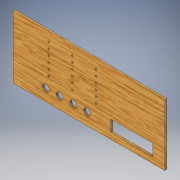
# Autodesk Inventor part: wooden-panel
Saved by Autodesk Inventor 2019.2 (Build 232265000, 265)
## iProperties
Created: 2020-05-18
Part Number: wooden-panel
Material: Laminated Veneer Lumber
Document SubType Name: Modeling
Designer: Johansson
Density: 0.51 g/cm^3
Appearance: Plywood - New
Author: Johansson
Autodesk Inventor part; units mm, degrees
ref_plane "YZ Plane" through (0, 0, 0) normal (1, 0, 0) x (0, 1, 0)
ref_plane "XZ Plane" through (0, 0, 0) normal (0, 1, 0) x (-1, 0, 0)
ref_plane "XY Plane" through (0, 0, 0) normal (0, 0, 1) x (1, 0, 0)
sketch "Sketch1" plane through (0, 0, 0) normal (0, 0, 1) x (1, 0, 0)
  line L0 (0, 0) -> (640, 0)
  line L1 (640, 0) -> (640, 260)
  line L2 (640, 260) -> (0, 265)
  line L3 (0, 265) -> (0, 0)
  dimension "d0" = 640
  dimension "d1" = 260
  dimension "d2" = 265
  constraints: 8 end point, 1 horizontal, 1 parallel, 1 perpendicular
  measures "d0" distance of L0.start L0.end
  measures "d1" distance of L0.end L1.end
  measures "d2" distance of L2.end L0.start
extrude "Extrusion1" add sketch "Sketch1" along normal blind 8
sketch "Sketch2" plane through (0, 0, 8) normal (0, 0, 1) x (1, 0, 0)
  line L0 (412, 75) -> (590, 75)
  line L1 (590, 75) -> (590, 25)
  line L2 (590, 25) -> (412, 25)
  line L3 (412, 25) -> (412, 75)
  line L4 (640, 0) -> (640, 260) projected
  line L5 (0, 0) -> (640, 0) projected
  dimension "d5" = 178
  dimension "d6" = 50
  dimension "d7" = 50
  dimension "d8" = 25
  constraints: 8 end point, 2 parallel, 1 horizontal, 1 perpendicular
  measures "d5" distance of L1.end L2.end
  measures "d6" distance of L0.end L1.end
  measures "d7" distance between parallel lines of L1 L4
  measures "d8" distance between parallel lines of L5 L2
extrude "Extrusion2" cut sketch "Sketch2" against normal up to next
sketch "Sketch3" plane through (0, 0, 8) normal (0, 0, 1) x (1, 0, 0)
  circle A0 centre (150, 100) radius 4
  line L0 (150, 314.3416) -> (150, 72.5342) construction
  line L1 (590, 75) -> (590, 25) projected
  line L2 (412, 75) -> (590, 75) projected
  line L3 (0, 265) -> (0, 0) projected
  dimension "d11" = 8
  dimension "d13" = 25
  dimension "d36" = 150
  constraints: 2 end point, 1 centre point, 1 point on line, 1 vertical
  measures "d11" diameter of A0
  measures "d13" distance from line of L2 A0.centre
  measures "d36" distance between parallel lines of L3 L0
extrude "Extrusion3" cut sketch "Sketch3" against normal up to next
sketch "Sketch5" plane through (0, 0, 8) normal (0, 0, 1) x (1, 0, 0)
  line L0 (481.6603, 50) -> (142.3397, 50) construction
  line L1 (205.9181, 75) -> (315.9941, 75) construction
  line L2 (319.7898, 25) -> (246.2477, 25) construction
  line L3 (590, 25) -> (412, 25) projected
  line L4 (412, 75) -> (590, 75) projected
  circle A0 centre (312, 50) radius 14.5
  line L5 (412, 25) -> (412, 75) projected
  point P0 (0, 0)
  dimension "d26" = 29
  dimension "d27" = 100
  constraints: 6 end point, 3 horizontal, 2 collinear, 2 midpoint, 1 centre point, 1 other
  measures "d26" diameter of A0
  measures "d27" distance from line of A0.centre L5
extrude "Extrusion5" cut sketch "Sketch5" against normal up to next
pattern_linear "Rectangular Pattern3" count 4 spacing 58 along (-1, 0, 0) of "Extrusion5"
pattern_linear "Rectangular Pattern4" count 3 spacing 100 along (1, 0, 0) count 6 spacing 25 along (0, 1, 0) of "Extrusion3"
equation "\"d0\" = l_panel"
equation "\"d1\" = wr_panel"
equation "\"d2\" = wl_panel"
equation "\"d3\" = t_panel"
equation "\"d5\" = l_stereo"
equation "\"d6\" = w_stereo"
equation "\"d7\" = d6"
equation "\"d8\" = 0.5 * d7"
equation "\"d9\" = t_panel"
equation "\"d11\" = r_button"
equation "\"d13\" = l_buttontobutton"
equation "\"d36\" = 3 * l_label"
equation "\"d14\" = t_panel"
equation "\"d26\" = r_usboutlet"
equation "\"d27\" = 2 * w_stereo"
equation "\"d28\" = t_panel"
equation "\"d32\" = 2 * r_usboutlet"
equation "\"d39\" = l_label + 2 * l_buttontobutton"
equation "\"d42\" = l_buttontobutton"
equation "\"l_panel\" = 640"
equation "\"wl_panel\" = 265"
equation "\"wr_panel\" = 260"
equation "\"t_panel\" = 8"
equation "\"r_button\" = 8"
equation "\"l_stereo\" = 178"
equation "\"d_stereo\" = 177"
equation "\"w_stereo\" = 50"
equation "\"w_label\" = 15"
equation "\"ro_labelscrew\" = 5"
equation "\"r_labelscrew\" = 2.5"
equation "\"l_buttontobutton\" = 25"
equation "\"r_usboutlet\" = 29"
equation "\"l_fastener_button\" = 19"
equation "\"l_label\" = 50"
body "Solid1"
